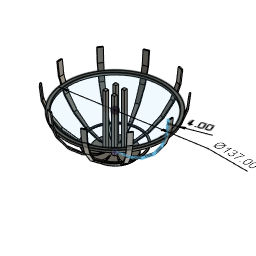
Bol skelet v4 (Autodesk Fusion 360 design; units mm, degrees)
Autodesk Fusion 360 part; units mm, degrees
sketch "Sketch2" plane through (0, 0, 0) normal (0, 0, 1) x (1, 0, 0)
  circle A0 centre (0, 0) radius 25
  dimension "d2" = 50
  constraint coincident A0.centre origin
  measures "d2" diameter of A0
extrude "Extrude1" add sketch "Sketch2" along normal blind 3 makes body 1
ref_plane "WorkPlane1" through (0, 0, 0) normal (0, 1, 0) x (0, 0, 1)
sketch "Sketch3" plane through (0, 0, 0) normal (0, 1, 0) x (1, 0, 0)
  line L0 (73.5, -75) -> (75, -75)
  line L1 (0, -1.5) -> (0, 0)
  line L2 (0, 0) -> (19.8294, -2.6067)
  line L3 (19.8294, -2.6067) -> (38.2071, -10.4972)
  line L4 (38.2071, -10.4972) -> (53.9153, -22.8767)
  line L5 (53.9153, -22.8767) -> (65.784, -38.9744)
  line L6 (65.784, -38.9744) -> (72.9643, -57.641)
  line L7 (72.9643, -57.641) -> (75, -75)
  line L8 (75, -75) -> (73.5, -75)
  line L9 (73.5, -75) -> (72.4825, -66.3238)
  line L10 (72.4825, -66.3238) -> (71.465, -57.6476)
  line L11 (71.465, -57.6476) -> (64.5414, -39.6482)
  line L12 (64.5414, -39.6482) -> (52.9005, -23.8595)
  line L13 (52.9005, -23.8595) -> (37.4854, -11.7109)
  line L14 (37.4854, -11.7109) -> (19.7502, -4.0963)
  line L15 (19.7502, -4.0963) -> (0, -1.5)
  dimension "d18" = 20
  dimension "d19" = 20
  dimension "d20" = 20
  dimension "d21" = 20
  dimension "d22" = 20
  dimension "d23" = 1.5
  dimension "d24" = 1.5
  dimension "d25" = 1.4
  dimension "d26" = 1.4
  dimension "d27" = 1.4
  constraint coincident L1.end L2.start
  constraint perpendicular L0 L1
  constraint parallel L7 L9
  constraint parallel L7 L10
  constraint parallel L6 L11
  constraint parallel L5 L12
  constraint parallel L4 L13
  constraint parallel L2 L15
  constraint parallel L3 L14
  measures "d18" distance of L1.end L2.end
  measures "d19" distance of L2.end L3.end
  measures "d20" distance of L3.end L4.end
  measures "d21" distance of L4.end L5.end
  measures "d22" distance of L5.end L6.end
  measures "d23" distance of L0.end L0.start
  measures "d24" distance of L1.end L1.start
  measures "d25" distance of L4 L13
  measures "d26" distance of L5 L12
  measures "d27" distance of L3 L14
revolve "Revolve3" add sketch "Sketch3" angle 5 about axis through (0, 0, 1.75) along (0, 0, 1) bodies 1
pattern_circular "C-Pattern1" count 10 over 360 about axis through (0, 0, 1.75) along (0, 0, 1) of bodies 1 makes body 2 at (55.7137, 48.4312, 69.2137) makes body 3 at (22.8121, 70.2083, 69.2137) makes body 4 at (-28.8443, 67.953, 69.2137) makes body 5 at (-63.2773, 38.0208, 69.2137) makes body 6 at (-73.8214, 0, 69.2137) makes body 7 at (-55.7137, -48.4312, 69.2137) makes body 8 at (-22.8121, -70.2083, 69.2137) makes body 9 at (22.8121, -70.2083, 69.2137) makes body 10 at (63.2773, -38.0208, 69.2137)
ref_plane "WorkPlane2" through (0, 0, 5) normal (0, 0, 1) x (1, 0, 0)
ref_plane "WorkPlane3" through (0, 0, 10) normal (0, 0, 1) x (1, 0, 0)
sketch "Sketch5" plane through (0, 0, 10) normal (0, 0, 1) x (1, 0, 0)
  circle A0 centre (0, 0) radius 35
  circle A1 centre (0, 0) radius 33
  dimension "d35" = 70
  dimension "d36" = 66
  constraint coincident A0.centre A1.centre
  constraint concentric A0 A1
  measures "d35" diameter of A0
  measures "d36" diameter of A1
extrude "Extrude2" add sketch "Sketch5" along normal blind 1 bodies 1 2 3 4 5 6 7 8 9 10
sketch "Sketch6" plane through (0, 0, 0) normal (0, 0, 1) x (1, 0, 0)
  line L0 (-8, 9) -> (-4, 9)
  line L1 (-4, 9) -> (-4, 5)
  line L2 (-4, 5) -> (-8, 5)
  line L3 (-8, 5) -> (-8, 9)
  line L4 (4, -5) -> (8, -5)
  line L5 (8, -5) -> (8, -9)
  line L6 (8, -9) -> (4, -9)
  line L7 (4, -9) -> (4, -5)
  line L8 (0, 0) -> (-8, 0)
  line L9 (-8, -9) -> (-4, -9)
  line L10 (-8, -5) -> (-8, -9)
  line L11 (-4, -9) -> (-4, -5)
  line L12 (-4, -5) -> (-8, -5)
  line L13 (4, 5) -> (8, 5)
  line L14 (8, 5) -> (8, 9)
  line L15 (8, 9) -> (4, 9)
  line L16 (4, 9) -> (4, 5)
  dimension "d39" = 4
  dimension "d40" = 5
  dimension "d41" = 4
  dimension "d42" = 4
  dimension "d43" = 5
  dimension "d44" = 4
  constraint horizontal L0
  constraint vertical L1
  constraint horizontal L2
  constraint vertical L3
  constraint horizontal L4
  constraint vertical L5
  constraint horizontal L6
  constraint vertical L7
  constraint coincident L8.start origin
  constraint horizontal L8
  constraint symmetric L0.start L8 L9.start
  constraint symmetric L0.end L8 L9.end
  constraint symmetric L1.end L8 L11.end
  constraint symmetric L2.end L8 L10.start
  constraint symmetric L4.start L8 L13.start
  constraint symmetric L4.end L8 L13.end
  constraint symmetric L5.end L8 L14.end
  constraint symmetric L6.end L8 L15.end
  measures "d39" distance of L8.start L1
  measures "d40" distance of L2 L8.start
  measures "d41" distance of L4.start L4.end
  measures "d42" distance of L4.start L6.end
  measures "d43" distance of L8.start L4
  measures "d44" distance of L8.start L7
extrude "Extrude3" add sketch "Sketch6" along normal blind 75 bodies 1
ref_plane "WorkPlane4" through (0, 0, 50) normal (0, 0, 1) x (1, 0, 0)
sketch "Sketch7" plane through (0, 0, 50) normal (0, 0, 1) x (1, 0, 0)
  circle A0 centre (0, 0) radius 68.5
  circle A1 centre (0, 0) radius 64.5
  dimension "d48" = 137
  dimension "d49" = 4
  constraint coincident A0.centre A1.centre
  constraint concentric A0 A1
  measures "d48" diameter of A0
  measures "d49" distance of A0 A1
extrude "Extrude4" add sketch "Sketch7" against normal blind 3 bodies 1
